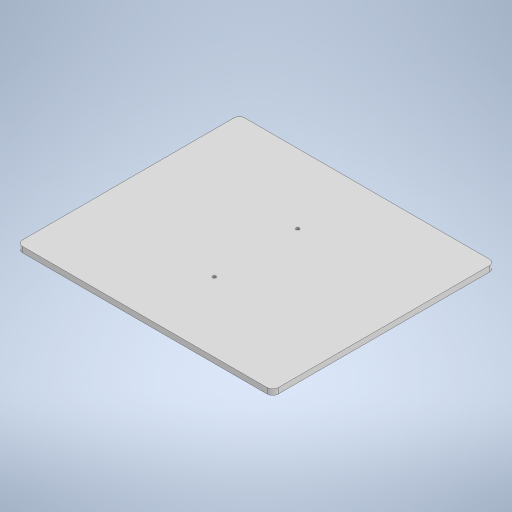
# Autodesk Inventor part: Pedana
Saved by Autodesk Inventor 2024 (Build 280153000, 153)
## iProperties
Created: 2023-11-20
Part Number: Pedana
Material: Generico
Document SubType Name: Modeling
Designer: Leonardo
Density: 1 g/cm^3
Appearance: Default
Author: Leonardo
## iProperties of the stored document Pedana_Stampa 3D.ipt
Created: 2023-12-15
Part Number: Pedana_Stampa 3D
Material: Generico
Document SubType Name: Modeling
Designer: Leonardo
Density: 1 g/cm^3
Appearance: Default
Author: Leonardo
Autodesk Inventor part; units mm, degrees
ref_plane "YZ Plane" through (0, 0, 0) normal (1, 0, 0) x (0, 1, 0)
ref_plane "XZ Plane" through (0, 0, 0) normal (0, 1, 0) x (-1, 0, 0)
ref_plane "XY Plane" through (0, 0, 0) normal (0, 0, 1) x (1, 0, 0)
sketch "Schizzo3" plane through (0, 0, 0) normal (0, 1, 0) x (-1, 0, 0)
  circle A0 centre (0, 75) radius 2.75
  circle A1 centre (0, -75) radius 2.75
  line L0 (-230, 0) -> (-230, 100)
  line L1 (230, 100) -> (230, 0)
  line L2 (-230, 0) -> (-230, -100)
  line L3 (230, -100) -> (230, 0)
  line L4 (-230, 0) -> (-230, 190)
  line L5 (-220, 200) -> (220, 200)
  line L6 (230, 190) -> (230, 2)
  line L7 (-230, 0) -> (-230, -190)
  line L8 (-220, -200) -> (220, -200)
  line L9 (230, -190) -> (230, 0)
  arc A2 (228, 0) -> (230, 2) centre (228, 2) ccw
  arc A3 (230, 190) -> (220, 200) centre (220, 190) ccw
  arc A4 (220, -200) -> (230, -190) centre (220, -190) ccw
  arc A5 (-230, -190) -> (-220, -200) centre (-220, -190) ccw
  arc A6 (-220, 200) -> (-230, 190) centre (-220, 190) ccw
  point P0 (0, 0)
  point P1 (-230, 200)
  point P2 (-230, -200)
  dimension "d18" = 5.5
  dimension "d21" = 5.5
  dimension "d24" = 460
  dimension "d25" = 460
  dimension "d26" = 100
  dimension "d27" = 200
  dimension "d28" = 200
  dimension "d29" = 2
  dimension "d30" = 10
  constraints: 20 end point, 10 point on circle, 9 tangent, 7 centre point, 6 point on line, 4 parallel, 3 equal radius
  measures "d18" diameter of A0
  measures "d21" diameter of A1
  measures "d24" distance of L0.end L1.start
  measures "d25" distance of L3.start L2.end
  measures "d26" distance of L2.end L2.start
  measures "d27" distance of L4.start point (-230, 200)
  measures "d28" distance of point (-230, -200) L7.start
  measures "d29" radius of A2
  measures "d30" radius of A3
extrude "Estrusione3" add sketch "Schizzo3" along normal blind 10
